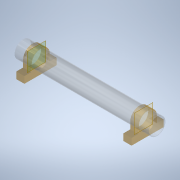
# Autodesk Inventor part: tubo transparente
Saved by Autodesk Inventor 2020 (Build 240168000, 168)
## iProperties
Created: 2020-02-18
Part Number: tubo transparente
Material: Vidrio
Document SubType Name: Modeling
Designer: PabloGod
Density: 2.18 g/cm^3
Appearance: Claro
Mass: 18.9537 g
Surface Area: 121.721 cm^2
Volume: 8.69436 cm^3
Author: PabloGod
Autodesk Inventor part; units mm, degrees
ref_plane "YZ Plane" through (0, 0, 0) normal (1, 0, 0) x (0, 1, 0)
ref_plane "XZ Plane" through (0, 0, 0) normal (0, 1, 0) x (-1, 0, 0)
ref_plane "XY Plane" through (0, 0, 0) normal (0, 0, 1) x (1, 0, 0)
sketch "Boceto1" plane through (0, 0, 0) normal (1, 0, 0) x (0, 1, 0)
  circle A0 centre (0, 0) radius 30
  circle A1 centre (0, 0) radius 31.5
  dimension "d0" = 60
  dimension "d1" = 63
  constraints: 2 centre point, 2 coincident
  measures "d0" diameter of A0
  measures "d1" diameter of A1
extrude "Extrusión1" add sketch "Boceto1" along normal blind 500
ref_plane "Plano de trabajo1" through (50, 0, 0) normal (-1, 0, 0) x (0, 0, 1)
ref_plane "Plano de trabajo2" through (450, 0, 0) normal (1, 0, 0) x (0, 0, -1)
sketch "Boceto2" plane through (50, 0, 0) normal (-1, 0, 0) x (0, 0, 1)
  circle A0 centre (0, 0) radius 32.5
  arc A1 (35, 0) -> (-35, 0) centre (0, 0) ccw
  line L0 (-35, 0) -> (-35, -25)
  line L1 (-35, -25) -> (-60, -25)
  line L2 (-60, -25) -> (-60, -50)
  line L3 (-60, -50) -> (60, -50)
  line L4 (60, -50) -> (60, -25)
  line L5 (60, -25) -> (35, -25)
  line L6 (35, -25) -> (35, 0)
  dimension "d6" = 65
  dimension "d7" = 70
  dimension "d8" = 25
  dimension "d9" = 25
  dimension "d10" = 25
  dimension "d11" = 120
  dimension "d12" = 25
  dimension "d13" = 25
  constraints: 14 end point, 3 perpendicular, 2 centre point, 2 coincident, 2 point on circle, 2 point on line, 2 tangent, 1 vertical
  measures "d6" diameter of A0
  measures "d7" diameter of A1
  measures "d8" distance of L0.start L0.end
  measures "d9" distance of L0.end L1.end
  measures "d10" distance of L1.end L2.end
  measures "d11" distance of L2.end L3.end
  measures "d12" distance of L3.end L4.end
  measures "d13" distance of L4.end L5.end
sketch "Boceto3" plane through (450, 0, 0) normal (1, 0, 0) x (0, 0, -1)
  circle A0 centre (0, 0) radius 32.5
  arc A1 (35, 0) -> (-35, 0) centre (0, 0) ccw
  line L0 (-35, 0) -> (-35, -25)
  line L1 (-35, -25) -> (-60, -25)
  line L2 (-60, -25) -> (-60, -50)
  line L3 (-60, -50) -> (60, -50)
  line L4 (60, -50) -> (60, -25)
  line L5 (60, -25) -> (35, -25)
  line L6 (35, -25) -> (35, 0)
  dimension "d14" = 65
  dimension "d15" = 70
  dimension "d16" = 25
  dimension "d17" = 25
  dimension "d18" = 25
  dimension "d19" = 120
  dimension "d20" = 25
  dimension "d21" = 25
  constraints: 14 end point, 3 perpendicular, 2 centre point, 2 coincident, 2 point on circle, 2 point on line, 2 tangent, 1 vertical
  measures "d14" diameter of A0
  measures "d15" diameter of A1
  measures "d16" distance of L0.start L0.end
  measures "d17" distance of L0.end L1.end
  measures "d18" distance of L1.end L2.end
  measures "d19" distance of L2.end L3.end
  measures "d20" distance of L3.end L4.end
  measures "d21" distance of L4.end L5.end
extrude "Extrusión2" add sketch "Boceto2" along normal mid plane 30
extrude "Extrusión3" add sketch "Boceto3" along normal mid plane 30
